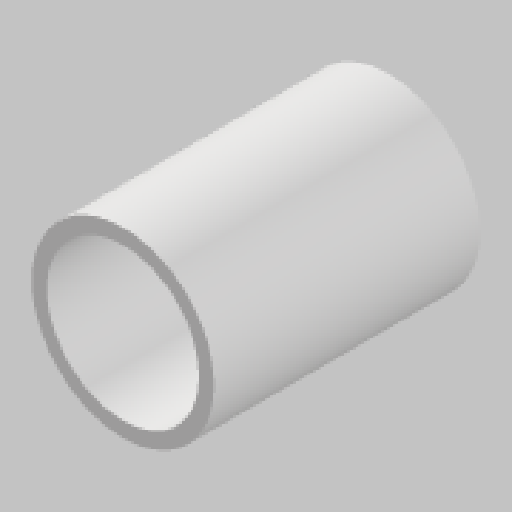
# Autodesk Inventor part: Buje verde
Saved by Autodesk Inventor 2024 (Build 280153000, 153)
## iProperties
Created: 2023-09-27
Part Number: Buje verde
Material: Generic
Document SubType Name: Modeling
Designer: ARViau
Density: 1 g/cm^3
Appearance: Default
Author: ARViau
Autodesk Inventor part; units mm, degrees
ref_plane "YZ Plane" through (0, 0, 0) normal (1, 0, 0) x (0, 1, 0)
ref_plane "XZ Plane" through (0, 0, 0) normal (0, 1, 0) x (-1, 0, 0)
ref_plane "XY Plane" through (0, 0, 0) normal (0, 0, 1) x (1, 0, 0)
sketch "Sketch1" plane through (0, 0, 0) normal (0, 0, 1) x (1, 0, 0)
  circle A0 centre (0, 0) radius 7.62 projected
  circle A1 centre (0, 0) radius 6.35 projected
extrude "Extrusion1" add sketch "Sketch1" along normal blind 22.225
body "Solid1"
